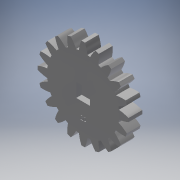
# Autodesk Inventor part: 20_teeth
Saved by Autodesk Inventor 2019 (Build 230136000, 136)
## iProperties
Created: 2020-02-24
Part Number: 20_teeth
Material: Steel
Document SubType Name: Modeling
Designer: Jeff
Categories: <?xml version="1.0" encoding="UTF-16"?> <MemberInstance><Categories><FamilyTemplate><FamilyTemplateParameter ValueType="xs:double" Id="1" ObjectReferenceKey="da_z" ObjectType="kUserParameterObject"/><FamilyTemplateParameter ValueType="xs:double" Id="2" ObjectReferenceKey="da_b" ObjectType="kUserParameterObject"/><FamilyTemplateParameter ValueType="xs:double" Id="3" ObjectReferenceKey="da_beta" ObjectType="kUserParameterObject"/><FamilyTemplateParameter ValueType="xs:double" Id="4" ObjectReferenceKey="da_da" ObjectType="kUserParameterObject"/><FamilyTemplateParameter ValueType="xs:double" Id="5" ObjectReferenceKey="da_aw" ObjectType="kUserParameterObject"/><FamilyTemplateParameter ValueType="xs:string" Id="6" ObjectReferenceKey="EAIAABAAAACIAQAAAAAAAIAAAAAAAAAA" ObjectType="83910656" SubObjectId="SurfaceGeometry"/></FamilyTemplate><ParamToTemplateMap><ParamToTemplate CategoryParameter="//CategoryParameter[@InternalName='046C89C9-8512-4d59-83FE-43B91F4F132A']" TemplateParameter="1"/><ParamToTemplate CategoryParameter="//CategoryParameter[@InternalName='2552DF32-E462-4b46-AEBF-C6C7768E72AC']" TemplateParameter="2"/><ParamToTemplate CategoryParameter="//CategoryParameter[@InternalName='C9EE641D-15FC-4fae-A226-E94C4372FDD7']" TemplateParameter="3"/><ParamToTemplate><ParamToTemplate CategoryParameter="//CategoryParameter[@InternalName='00B6519A-459B-49c7-AD84-2E56D39A5744']" ConstantValue="0.000000"/></ParamToTemplate><ParamToTemplate><ParamToTemplate CategoryParameter="//CategoryParameter[@InternalName='04B31F0E-C7A6-4894-AA32-9629BEFACF47']" ConstantValue="1.000000"/></ParamToTemplate><ParamToTemplate><ParamToTemplate CategoryParameter="//CategoryParameter[@InternalName='43CBEC2E-7847-49e7-A936-2F7889FCB2D9']" ConstantValue="0.250000"/></ParamToTemplate><ParamToTemplate><ParamToTemplate CategoryParameter="//CategoryParameter[@InternalName='B1EFC894-105D-4ebd-86BF-FA20ED196853']" ConstantValue="0.350000"/></ParamToTemplate><ParamToTemplate><ParamToTemplate CategoryParameter="//CategoryParameter[@InternalName='51175063-3D10-4879-93E8-6246FE8B403D']" ConstantValue="2060000000.000000"/></ParamToTemplate><ParamToTemplate><ParamToTemplate CategoryParameter="//CategoryParameter[@InternalName='A3A52E27-4454-46a9-B0BD-C932399B70AF']" ConstantValue="0.300000"/></ParamToTemplate><ParamToTemplate><ParamToTemplate CategoryParameter="//CategoryParameter[@InternalName='91B76062-C214-41d9-B1B9-14D2AB99603D']" ConstantValue="0.300000"/></ParamToTemplate><ParamToTemplate><ParamToTemplate CategoryParameter="//CategoryParameter[@InternalName='374E806E-8B8A-4dda-A9AA-1039D6500AD2']" ConstantValue="3.333333"/></ParamToTemplate><ParamToTemplate><ParamToTemplate CategoryParameter="//CategoryParameter[@InternalName='2D373A89-B862-43d6-8D0B-0CBF12AB9F6C']" ConstantValue="0.349066"/></ParamToTemplate><ParamToTemplate CategoryParameter="//CategoryParameter[@InternalName='37777632-D6A2-4fac-9D53-DB8ACD95C989']" TemplateParameter="4"/><ParamToTemplate CategoryParameter="//CategoryParameter[@InternalName='FD1017F1-B727-4f7e-9707-0F86F1FF9423']" TemplateParameter="5"/><ParamToTemplate><ParamToTemplate CategoryParameter="//CategoryParameter[@InternalName='9E1B4470-B2D3-4ff1-B813-535BB4CDF51A']" ConstantValue="3520000.000000"/></ParamToTemplate><ParamToTemplate><ParamToTemplate CategoryParameter="//CategoryParameter[@InternalName='F8452263-BFF6-458c-9FB1-07C4B99E95CD']" ConstantValue="11400000.000000"/></ParamToTemplate><ParamToTemplate><ParamToTemplate CategoryParameter="//CategoryParameter[@InternalName='3E3BB259-FD49-497f-8171-6EBC954A3479']" ConstantValue="2.000000"/></ParamToTemplate><ParamToTemplate CategoryParameter="//CategoryParameter[@InternalName='27C3BAF2-7550-4e4b-AE2C-0DB134B7D9B7']" TemplateParameter="6"/></ParamToTemplateMap><Category DisplayName="Gear" InternalName="DC85795E-93AB-48d5-8EEE-5A27447B64BD" Mnemonic="Gear"><CategoryParameter DisplayName="z" InternalName="046C89C9-8512-4d59-83FE-43B91F4F132A" Mnemonic="z"/><CategoryParameter DisplayName="b" InternalName="2552DF32-E462-4b46-AEBF-C6C7768E72AC" Mnemonic="b"/><CategoryParameter DisplayName="||b|" InternalName="C9EE641D-15FC-4fae-A226-E94C4372FDD7" Mnemonic="beta"/><CategoryParameter DisplayName="x" InternalName="00B6519A-459B-49c7-AD84-2E56D39A5744" Mnemonic="x"/><CategoryParameter DisplayName="a*" InternalName="04B31F0E-C7A6-4894-AA32-9629BEFACF47" Mnemonic="a"/><CategoryParameter DisplayName="c*" InternalName="43CBEC2E-7847-49e7-A936-2F7889FCB2D9" Mnemonic="c"/><CategoryParameter DisplayName="r|.f|*" InternalName="B1EFC894-105D-4ebd-86BF-FA20ED196853" Mnemonic="rf"/><CategoryParameter DisplayName="E" InternalName="51175063-3D10-4879-93E8-6246FE8B403D" Mnemonic="E"/><CategoryParameter DisplayName="||m|" InternalName="A3A52E27-4454-46a9-B0BD-C932399B70AF" Mnemonic="mi"/><Category DisplayName="SpurGear" InternalName="26C5A22E-A91E-4dfd-A3B3-23CCAFAE1764" Mnemonic="SpurGear"><CategoryParameter DisplayName="m" InternalName="91B76062-C214-41d9-B1B9-14D2AB99603D" Mnemonic="m"/><CategoryParameter DisplayName="P" InternalName="374E806E-8B8A-4dda-A9AA-1039D6500AD2" Mnemonic="PP"/><CategoryParameter DisplayName="||a|" InternalName="2D373A89-B862-43d6-8D0B-0CBF12AB9F6C" Mnemonic="alpha"/><CategoryParameter DisplayName="d|.a|" InternalName="37777632-D6A2-4fac-9D53-DB8ACD95C989" Mnemonic="da"/><CategoryParameter DisplayName="a|.w|" InternalName="FD1017F1-B727-4f7e-9707-0F86F1FF9423" Mnemonic="aw"/><CategoryParameter DisplayName="||s||.Flim|" InternalName="9E1B4470-B2D3-4ff1-B813-535BB4CDF51A" Mnemonic="sFlim"/><CategoryParameter DisplayName="||s||.Hlim|" InternalName="F8452263-BFF6-458c-9FB1-07C4B99E95CD" Mnemonic="sHlim"/><CategoryParameter DisplayName="type" InternalName="3E3BB259-FD49-497f-8171-6EBC954A3479" Mnemonic="type"/><CategoryParameter DisplayName="PitchDiameter" InternalName="27C3BAF2-7550-4e4b-AE2C-0DB134B7D9B7" Mnemonic="IDS_PITCHDIAM"/></Category></Category></Categories></MemberInstance>
Density: 1 g/cm^3
Appearance: Steel
CustomPartVersion: 1
Author: Jeff
Autodesk Inventor part; units mm, degrees
sketch "Sketch1" plane through (0, 0, 0) normal (0, 0, 1) x (1, 0, 0)
  circle A0 centre (0, 0) radius 33
  dimension "d0" = 66
  constraints: 1 centre point
  measures "d0" diameter of A0
extrude "Extrusion1" add sketch "Sketch1" along normal blind 10
ref_plane "Work Plane2" through (0, 0, 5) normal (0, 0, 1) x (1, 0, 0)
sketch "Sketch2" plane through (0, 0, 0) normal (0, 0, -1) x (-1, 0, 0)
  circle A0 centre (0, 0) radius 33 projected
  circle A1 centre (0, 0) radius 30
  dimension "d3" = 60
  constraints: 1 centre point, 1 coincident
  measures "d3" diameter of A1
surface extrude "Pitch Diameter" sketch "Sketch2" against normal through all shown no curves A1
ref_plane "Work Plane8" through (0, 0, 0) normal (0.9876883, 0.1564345, 0) x (0, 0, 1)
ref_plane "Work Plane9" through (0, 0, 0) normal (1, 0, 0) x (0, 1, 0)
spur gear teeth "Spur Gear" teeth 20 pitch diameter 60 tip diameter 66 root diameter 52.5 face width 10 start plane through (0, 0, 0) normal (0, 0, -1) x (-1, 0, 0)
sketch "Sketch3" plane through (0, 0, 10) normal (0, 0, 1) x (1, 0, 0)
  line L0 (-5, 5) -> (5, 5)
  line L1 (5, 5) -> (5, -5)
  line L2 (5, -5) -> (-5, -5)
  line L3 (-5, -5) -> (-5, 5)
  line L4 (-5, -20.534) -> (-5, -10.534) construction
  line L5 (-5, -10.534) -> (5, -10.534) construction
  line L6 (5, -10.534) -> (5, -20.534) construction
  line L7 (5, -20.534) -> (-5, -20.534) construction
  line L8 (-3.0854, -26.068) -> (-3.0854, -5)
  line L9 (-0.1823, -17.034) -> (-2.0324, -17.034)
  line L10 (-2.0324, -17.034) -> (-2.0324, -16.6086)
  spline S0 degree 2 poles (-2.0324, -16.6086) (-1.8331, -16.4214) (-1.4781, -16.0737) (-1.3079, -15.8865) knots 0 0 0 1 2 2 2
  spline S1 degree 2 poles (-1.3079, -15.8865) (-0.9652, -15.5097) (-0.7147, -15.0575) (-0.7147, -14.8168) knots 0 0 0 1 2 2 2
  spline S2 degree 2 poles (-0.7147, -14.8168) (-0.7147, -14.6904) (-0.7925, -14.5008) (-0.863, -14.44) knots 0 0 0 1 2 2 2
  spline S3 degree 2 poles (-0.863, -14.44) (-0.9335, -14.3792) (-1.1183, -14.3185) (-1.2301, -14.3185) knots 0 0 0 1 2 2 2
  spline S4 degree 2 poles (-1.2301, -14.3185) (-1.3371, -14.3185) (-1.5559, -14.3719) (-1.6556, -14.4133) knots 0 0 0 1 2 2 2
  spline S5 degree 2 poles (-1.6556, -14.4133) (-1.7407, -14.4473) (-1.8987, -14.5446) (-1.9473, -14.5786) knots 0 0 0 1 2 2 2
  line L11 (-1.9473, -14.5786) -> (-1.9692, -14.5786)
  line L12 (-1.9692, -14.5786) -> (-1.9692, -14.1507)
  spline S6 degree 2 poles (-1.9692, -14.1507) (-1.8452, -14.0899) (-1.4003, -13.9708) (-1.201, -13.9708) knots 0 0 0 1 2 2 2
  spline S7 degree 2 poles (-1.201, -13.9708) (-0.7804, -13.9708) (-0.3063, -14.4157) (-0.3063, -14.795) knots 0 0 0 1 2 2 2
  spline S8 degree 2 poles (-0.3063, -14.795) (-0.3063, -14.9724) (-0.389, -15.269) (-0.4619, -15.3954) knots 0 0 0 1 2 2 2
  spline S9 degree 2 poles (-0.4619, -15.3954) (-0.5348, -15.5267) (-0.7464, -15.7844) (-0.863, -15.9084) knots 0 0 0 1 2 2 2
  spline S10 degree 2 poles (-0.863, -15.9084) (-1.0527, -16.1151) (-1.517, -16.5575) (-1.6556, -16.6864) knots 0 0 0 1 2 2 2
  line L13 (-1.6556, -16.6864) -> (-0.1823, -16.6864)
  line L14 (-0.1823, -16.6864) -> (-0.1823, -17.034)
  spline S11 degree 2 poles (2.0859, -15.534) (2.0859, -16.3412) (1.6167, -17.0972) (1.128, -17.0972) knots 0 0 0 1 2 2 2
  spline S12 degree 2 poles (1.128, -17.0972) (0.6321, -17.0972) (0.1677, -16.3266) (0.1677, -15.5365) knots 0 0 0 1 2 2 2
  spline S13 degree 2 poles (0.1677, -15.5365) (0.1677, -14.7245) (0.637, -13.9732) (1.128, -13.9732) knots 0 0 0 1 2 2 2
  spline S14 degree 2 poles (1.128, -13.9732) (1.6216, -13.9732) (2.0859, -14.7512) (2.0859, -15.534) knots 0 0 0 1 2 2 2
  spline S15 degree 2 poles (1.5705, -16.4481) (1.6288, -16.2998) (1.6775, -15.8428) (1.6775, -15.534) knots 0 0 0 1 2 2 2
  spline S16 degree 2 poles (1.6775, -15.534) (1.6775, -15.2253) (1.6288, -14.7707) (1.5681, -14.6175) knots 0 0 0 1 2 2 2
  spline S17 degree 2 poles (1.5681, -14.6175) (1.5073, -14.4643) (1.2958, -14.3063) (1.128, -14.3063) knots 0 0 0 1 2 2 2
  spline S18 degree 2 poles (1.128, -14.3063) (0.9603, -14.3063) (0.7439, -14.4643) (0.6807, -14.6224) knots 0 0 0 1 2 2 2
  spline S19 degree 2 poles (0.6807, -14.6224) (0.6199, -14.7755) (0.5762, -15.2423) (0.5762, -15.5365) knots 0 0 0 1 2 2 2
  spline S20 degree 2 poles (0.5762, -15.5365) (0.5762, -15.8525) (0.6151, -16.2755) (0.6783, -16.4408) knots 0 0 0 1 2 2 2
  spline S21 degree 2 poles (0.6783, -16.4408) (0.7366, -16.5964) (0.953, -16.7642) (1.128, -16.7642) knots 0 0 0 1 2 2 2
  spline S22 degree 2 poles (1.128, -16.7642) (1.2934, -16.7642) (1.5097, -16.6061) (1.5705, -16.4481) knots 0 0 0 1 2 2 2
  point P0 (0, 0)
  point P1 (0, 5)
  point P2 (5, 0)
  point P3 (0, -10.534)
  point P4 (-5, -15.534)
  point P5 (-3.0854, -15.534)
  dimension "d49" = 10
  dimension "d50" = 10
  dimension "d56" = 10
  dimension "d57" = 10
  constraints: 10 end point, 5 midpoint, 2 horizontal, 2 horizontal alignment, 2 parallel, 2 perpendicular, 1 point on line, 1 vertical alignment, 2 other
  measures "d49" distance of L1.end L2.end
  measures "d50" distance of L0.end L1.end
  measures "d56" distance between parallel lines of L6 L4
  measures "d57" distance between parallel lines of L5 L7
extrude "Extrusion2" cut sketch "Sketch3" against normal blind 4
sketch "Sketch4" plane through (0, 0, 0) normal (0, 0, -1) x (-1, 0, 0)
  circle A0 centre (0, 0) radius 7.5
  dimension "d53" = 15
  constraints: 1 centre point, 1 coincident
  measures "d53" diameter of A0
extrude "Extrusion3" cut sketch "Sketch4" against normal blind 4
equation "\"d0\" = da_da"
equation "\"d1\" = da_b"
equation "\"d3\" = da_dw"
equation "\"d16\" = da_aw"
equation "\"d43\" = da_aw"
equation "\"d46\" = da_aw"
equation "\"da_da\" = 66"
equation "\"da_b\" = 10"
equation "\"da_dw\" = 60"
equation "\"da_aw\" = 45"
body "Solid1"
body "Srf1"
